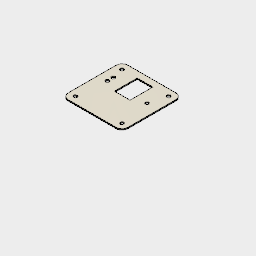
ATTEMP-FACEPLATE (Autodesk Fusion 360 design; units mm, degrees)
Autodesk Fusion 360 part; units mm, degrees
sketch "Sketch1" plane through (0, 45.8, 0) normal (0, 1, 0) x (-1, 0, 0)
  arc A0 (-42.5, 47.5) -> (-47.5, 42.5) centre (-42.5, 42.5) ccw
  line L0 (-47.5, 42.5) -> (-47.5, 2.5)
  arc A1 (-47.5, 2.5) -> (-42.5, -2.5) centre (-42.5, 2.5) ccw
  line L1 (-42.5, -2.5) -> (-2.5, -2.5)
  arc A2 (-2.5, -2.5) -> (2.5, 2.5) centre (-2.5, 2.5) ccw
  line L2 (2.5, 2.5) -> (2.5, 42.5)
  arc A3 (2.5, 42.5) -> (-2.5, 47.5) centre (-2.5, 42.5) ccw
  line L3 (-2.5, 47.5) -> (-42.5, 47.5)
  circle A4 centre (-3, 42) radius 1.5
  circle A5 centre (-3, 3) radius 1.5
  circle A6 centre (-42, 42) radius 1.5
  circle A7 centre (-42, 3) radius 1.5
  arc A8 (-4, 8.5) -> (-8.5, 4) centre (-4, 4) ccw
  line L4 (-8.5, 4) -> (-8.5, 0)
  line L5 (-8.5, 0) -> (-36.5, 0)
  line L6 (-36.5, 0) -> (-36.5, 4)
  arc A9 (-36.5, 4) -> (-41, 8.5) centre (-41, 4) ccw
  line L7 (-41, 8.5) -> (-45, 8.5)
  line L8 (-45, 8.5) -> (-45, 36.5)
  line L9 (-45, 36.5) -> (-41, 36.5)
  arc A10 (-41, 36.5) -> (-36.5, 41) centre (-41, 41) ccw
  line L10 (-36.5, 41) -> (-36.5, 45)
  line L11 (-8.5, 45) -> (-8.5, 41)
  arc A11 (-8.5, 41) -> (-4, 36.5) centre (-4, 41) ccw
  line L12 (-4, 36.5) -> (0, 36.5)
  line L13 (0, 36.5) -> (0, 8.5)
  line L14 (0, 8.5) -> (-4, 8.5)
  line L15 (2.5, 2.5) -> (2.5, 42.5)
  line L16 (-42.5, -2.5) -> (-2.5, -2.5)
  arc A12 (-2.5, -2.5) -> (2.5, 2.5) centre (-2.5, 2.5) ccw
  arc A13 (-47.5, 2.5) -> (-42.5, -2.5) centre (-42.5, 2.5) ccw
  line L17 (-47.5, 42.5) -> (-47.5, 2.5)
  arc A14 (-42.5, 47.5) -> (-47.5, 42.5) centre (-42.5, 42.5) ccw
  line L18 (-2.5, 47.5) -> (-42.5, 47.5)
  arc A15 (2.5, 42.5) -> (-2.5, 47.5) centre (-2.5, 42.5) ccw
  line L19 (-15.6736, 2.9508) -> (-28.6736, 2.9508)
  line L20 (-28.6736, 2.9508) -> (-28.6736, 21.9508)
  line L21 (-28.6736, 21.9508) -> (-15.6736, 21.9508)
  line L22 (-15.6736, 21.9508) -> (-15.6736, 2.9508)
  circle A16 centre (-42, 42) radius 1.5
  circle A17 centre (-42, 3) radius 1.5
  circle A18 centre (-3, 3) radius 1.5
  circle A19 centre (-3, 42) radius 1.5
  point P0 (-15.6736, 2.9508)
  point P1 (-28.6736, 21.9508)
  dimension "d187" = 3
  dimension "d188" = 3
  dimension "d189" = 3
  measures "d187" diameter of A16
  measures "d188" diameter of A18
  measures "d189" diameter of A19
extrude "Extrude1" add sketch "Sketch1" along normal blind 1
sketch "Sketch2" plane through (0, 46.8, 0) normal (0, 1, 0) x (-1, 0, 0)
  circle A0 centre (-3, 3) radius 1.5
  circle A1 centre (-42, 3) radius 1.5
  circle A2 centre (-42, 42) radius 1.5
  line L0 (-28.6736, 21.9508) -> (-15.6736, 21.9508)
  line L1 (-15.6736, 21.9508) -> (-15.6736, 2.9508)
  line L2 (-15.6736, 2.9508) -> (-28.6736, 2.9508)
  line L3 (-28.6736, 2.9508) -> (-28.6736, 21.9508)
  circle A3 centre (-3, 42) radius 1.5
  arc A4 (2.5, 42.5) -> (-2.5, 47.5) centre (-2.5, 42.5) ccw
  line L4 (-2.5, 47.5) -> (-42.5, 47.5)
  arc A5 (-42.5, 47.5) -> (-47.5, 42.5) centre (-42.5, 42.5) ccw
  line L5 (-47.5, 42.5) -> (-47.5, 2.5)
  arc A6 (-47.5, 2.5) -> (-42.5, -2.5) centre (-42.5, 2.5) ccw
  line L6 (-42.5, -2.5) -> (-2.5, -2.5)
  arc A7 (-2.5, -2.5) -> (2.5, 2.5) centre (-2.5, 2.5) ccw
  line L7 (2.5, 2.5) -> (2.5, 42.5)
  circle A8 centre (-5.25, 12.5) radius 1.5
  circle A9 centre (-5.25, 12.5) radius 1.5
  circle A10 centre (-5.25, 17.5) radius 1.5
  circle A11 centre (-5.25, 17.5) radius 1.5
  circle A12 centre (-38, 17) radius 1.5
  circle A13 centre (-38, 17) radius 1.5
sketch "Sketch3" plane through (0, 46.8, 0) normal (0, 1, 0) x (-1, 0, 0)
  circle A0 centre (-3, 3) radius 1.5
  circle A1 centre (-42, 3) radius 1.5
  circle A2 centre (-42, 42) radius 1.5
  line L0 (-28.6736, 21.9508) -> (-15.6736, 21.9508)
  line L1 (-15.6736, 21.9508) -> (-15.6736, 2.9508)
  line L2 (-15.6736, 2.9508) -> (-28.6736, 2.9508)
  line L3 (-28.6736, 2.9508) -> (-28.6736, 21.9508)
  circle A3 centre (-3, 42) radius 1.5
  arc A4 (2.5, 42.5) -> (-2.5, 47.5) centre (-2.5, 42.5) ccw
  line L4 (-2.5, 47.5) -> (-42.5, 47.5)
  arc A5 (-42.5, 47.5) -> (-47.5, 42.5) centre (-42.5, 42.5) ccw
  line L5 (-47.5, 42.5) -> (-47.5, 2.5)
  arc A6 (-47.5, 2.5) -> (-42.5, -2.5) centre (-42.5, 2.5) ccw
  line L6 (-42.5, -2.5) -> (-2.5, -2.5)
  arc A7 (-2.5, -2.5) -> (2.5, 2.5) centre (-2.5, 2.5) ccw
  line L7 (2.5, 2.5) -> (2.5, 42.5)
  circle A8 centre (-5.25, 12.5) radius 1.5
  circle A9 centre (-5.25, 12.5) radius 1.5
  circle A10 centre (-5.25, 12.5) radius 1.5
  circle A11 centre (-5.25, 17.5) radius 1.5
  circle A12 centre (-38, 17) radius 1.5
  point P0 (-5.25, 12.5)
  point P1 (-5.25, 17.5)
  point P2 (-6.75, 17.5)
  point P3 (-38, 17)
  point P4 (-39.5, 17)
sketch "Sketch4" plane through (0, 46.8, 0) normal (0, 1, 0) x (-1, 0, 0)
  circle A0 centre (-3, 3) radius 1.5
  circle A1 centre (-42, 3) radius 1.5
  circle A2 centre (-42, 42) radius 1.5
  line L0 (-28.6736, 21.9508) -> (-15.6736, 21.9508)
  line L1 (-15.6736, 21.9508) -> (-15.6736, 2.9508)
  line L2 (-15.6736, 2.9508) -> (-28.6736, 2.9508)
  line L3 (-28.6736, 2.9508) -> (-28.6736, 21.9508)
  circle A3 centre (-3, 42) radius 1.5
  arc A4 (2.5, 42.5) -> (-2.5, 47.5) centre (-2.5, 42.5) ccw
  line L4 (-2.5, 47.5) -> (-42.5, 47.5)
  arc A5 (-42.5, 47.5) -> (-47.5, 42.5) centre (-42.5, 42.5) ccw
  line L5 (-47.5, 42.5) -> (-47.5, 2.5)
  arc A6 (-47.5, 2.5) -> (-42.5, -2.5) centre (-42.5, 2.5) ccw
  line L6 (-42.5, -2.5) -> (-2.5, -2.5)
  arc A7 (-2.5, -2.5) -> (2.5, 2.5) centre (-2.5, 2.5) ccw
  line L7 (2.5, 2.5) -> (2.5, 42.5)
extrude "Extrude2" cut sketch "Sketch3" sketch "Sketch2" against normal blind 4 contours A12 of sketch 2 contours A8 A9 | A10 A11
sketch "sketch 1931" plane through (0, 14.8, 0) normal (0, 1, 0) x (-1, 0, 0)
  circle A0 centre (-38, 17) radius 1.5
  circle A1 centre (-38, 17) radius 2.65
extrude "Extrude3" cut sketch "sketch 1931" against normal blind 4
sketch "sketch 1947" plane through (0, 14.8, 0) normal (0, 1, 0) x (-1, 0, 0)
  circle A0 centre (-5.25, 12.5) radius 1.5
  circle A1 centre (-5.25, 17.5) radius 1.5
  arc A2 (-3.2306, 17.5) -> (-7.2694, 17.5) centre (-5.25, 17.5) ccw
  line L0 (-7.2694, 17.5) -> (-7.2694, 12.5)
  arc A3 (-7.2694, 12.5) -> (-3.2306, 12.5) centre (-5.25, 12.5) ccw
  line L1 (-3.2306, 12.5) -> (-3.2306, 17.5)
extrude "Extrude4" cut sketch "sketch 1947" against normal blind 1
